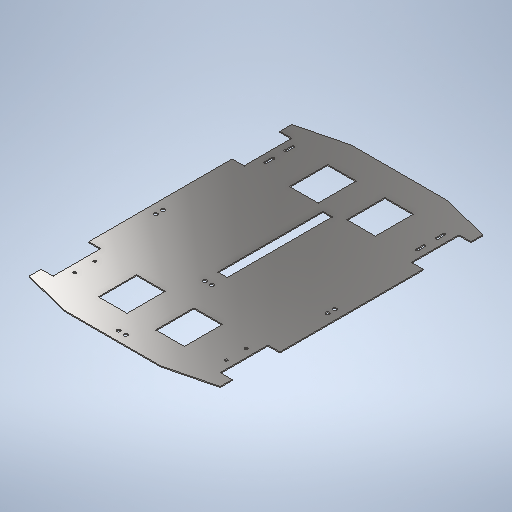
# Autodesk Inventor part: chassis
Saved by Autodesk Inventor 2026.1 (Build 301233020, 233B)
## iProperties
Created: 2026-01-22
Part Number: chassis
Material: Steel, Mild
Document SubType Name: Modeling
Designer: user
Density: 7.85 g/cm^3
Appearance: Semi-Polished
Mass: 3211.32 g
Surface Area: 4154.01 cm^2
Volume: 409.085 cm^3
Author: user
Autodesk Inventor part; units mm, degrees
ref_plane "YZ Plane" through (0, 0, 0) normal (1, 0, 0) x (0, 1, 0)
ref_plane "XZ Plane" through (0, 0, 0) normal (0, 1, 0) x (-1, 0, 0)
sketch "Sketch1" plane through (0, 0, 0) normal (0, 1, 0) x (-1, 0, 0)
  line L0 (-200, 300) -> (200, 300)
  line L1 (200, 300) -> (200, -300)
  line L2 (200, -300) -> (-200, -300)
  line L3 (-200, -300) -> (-200, 300)
  line L4 (-200, 300) -> (200, -300) construction
  line L5 (200, 300) -> (-200, -300) construction
  point P0 (0, 0)
  dimension "d0" = 400
  dimension "d1" = 600
  constraints: 12 end point, 2 midpoint, 2 parallel, 1 horizontal, 1 perpendicular
  measures "d0" distance of L1.end L2.end
  measures "d1" distance of L0.end L1.end
extrude "Extrusion1" add sketch "Sketch1" along normal blind 2
sketch "Sketch2" plane through (0, 2, 0) normal (0, 1, 0) x (1, 0, 0)
  line L0 (200, 300) -> (-200, 300) projected
  line L1 (-200, 300) -> (-200, 275)
  line L2 (-200, 300) -> (-200, -300) projected
  line L3 (-200, 300) -> (-100, 300)
  line L4 (-100, 300) -> (-200, 275)
  line L5 (-200, 275) -> (-200, 250)
  line L6 (-200, 250) -> (-175, 250)
  line L7 (-175, 250) -> (-175, 150)
  line L8 (-175, 150) -> (-200, 150)
  line L9 (-200, 250) -> (-200, 150)
  line L10 (0, 250) -> (0, 74.4907)
  line L11 (-155.9773, 0) -> (157.8952, 0)
  line L12 (-200, 300) -> (200, 300)
  line L13 (200, 300) -> (200, -300)
  line L14 (100, 300) -> (200, 275)
  line L15 (200, 250) -> (175, 250)
  line L16 (175, 250) -> (175, 150)
  line L17 (175, 150) -> (200, 150)
  line L18 (200, -300) -> (-200, -300)
  line L19 (-200, -300) -> (-200, -275)
  line L20 (-200, -300) -> (-100, -300)
  line L21 (-100, -300) -> (-200, -275)
  line L22 (-200, -275) -> (-200, -250)
  line L23 (-200, -250) -> (-175, -250)
  line L24 (-175, -250) -> (-175, -150)
  line L25 (-175, -150) -> (-200, -150)
  line L26 (-200, -250) -> (-200, -150)
  line L27 (175, -250) -> (175, -150)
  line L28 (175, -150) -> (200, -150)
  line L29 (200, -300) -> (200, 300)
  line L30 (200, -250) -> (175, -250)
  line L31 (100, -300) -> (200, -275)
  line L32 (-200, -300) -> (200, -300)
  point P0 (0, 0)
  dimension "d4" = 25
  dimension "d5" = 100
  dimension "d6" = 25
  dimension "d7" = 25
  dimension "d8" = 100
  constraints: 62 end point, 26 symmetric about line, 13 point on line, 3 perpendicular, 1 collinear, 1 horizontal, 1 vertical
  measures "d4" distance of L0.end L1.end
  measures "d5" distance of L0.end L3.end
  measures "d6" distance of L1.end L5.end
  measures "d7" distance of L5.end L6.end
  measures "d8" distance of L6.end L7.end
extrude "Extrusion2" cut sketch "Sketch2" against normal blind 2 contours L13 L14 L0 | L4 L1 L0 | L13 L17 L16 L15 | L6 L7 L8 L2 | L13 L30 L27 L28 | L25 L24 L23 L2 | L13 L18 L31 | L21 L18 L2
sketch "Sketch3" plane through (0, 2, 0) normal (0, 1, 0) x (1, 0, 0)
  line L0 (-175, 250) -> (-200, 250) projected
  line L1 (-175, 250) -> (-175, 200)
  line L2 (-175, 150) -> (-175, 250) projected
  line L3 (175, 250) -> (200, 250) projected
  line L4 (175, 250) -> (175, 200)
  line L5 (175, 250) -> (175, 150) projected
  line L6 (175, 200) -> (-175, 200)
  line L7 (-175, -150) -> (-175, -251.235)
  line L8 (-175, -251.235) -> (-175, -201.235)
  line L9 (-175, -150) -> (-175, -250) projected
  line L10 (-175, -201.235) -> (175, -201.235)
  line L11 (-175, 200) -> (-165, 200)
  line L12 (-165, 200) -> (-165, 227.5)
  line L13 (-165, 227.5) -> (-152, 227.5)
  line L14 (-152, 227.5) -> (-152, 172.5)
  line L15 (-152, 172.5) -> (-165, 172.5)
  line L16 (-165, 172.5) -> (-165, 200)
  line L17 (0, 46.6917) -> (0, -57.1112)
  line L18 (0, 0) -> (63.947, 0)
  line L19 (63.947, 0) -> (-44.9417, 0)
  line L20 (165, 200) -> (165, 227.5)
  line L21 (165, 227.5) -> (152, 227.5)
  line L22 (152, 227.5) -> (152, 172.5)
  line L23 (152, 172.5) -> (165, 172.5)
  line L24 (165, 172.5) -> (165, 200)
  line L25 (-165, -200) -> (-165, -227.5)
  line L26 (-165, -227.5) -> (-152, -227.5)
  line L27 (-152, -227.5) -> (-152, -172.5)
  line L28 (-152, -172.5) -> (-165, -172.5)
  line L29 (-165, -172.5) -> (-165, -200)
  line L30 (152, -227.5) -> (152, -172.5)
  line L31 (152, -172.5) -> (165, -172.5)
  line L32 (165, -172.5) -> (165, -200)
  line L33 (165, -200) -> (165, -227.5)
  line L34 (165, -227.5) -> (152, -227.5)
  line L35 (-165, 227.5) -> (-158.5, 227.5)
  line L36 (-158.5, 227.5) -> (-158.5, 221)
  circle A0 centre (-158.5, 221) radius 2.5
  circle A1 centre (-158.5, 179) radius 2.5
  circle A2 centre (158.5, 221) radius 2.5
  circle A3 centre (158.5, 179) radius 2.5
  circle A4 centre (158.5, -179) radius 2.5
  circle A5 centre (158.5, -221) radius 2.5
  circle A6 centre (-158.5, -179) radius 3
  circle A7 centre (-158.5, -221) radius 3
  dimension "d11" = 50
  dimension "d12" = 50
  dimension "d13" = 50
  dimension "d14" = 10
  dimension "d15" = 27.5
  dimension "d16" = 13
  dimension "d17" = 55
  dimension "d18" = 6.5
  dimension "d19" = 5
  dimension "d110" = 6
  dimension "d111" = 6
  constraints: 64 end point, 20 symmetric about line, 8 centre point, 8 perpendicular, 7 point on line, 3 midpoint, 2 vertical, 1 coincident, 1 horizontal, 5 other
  measures "d11" distance of L0.start L1.end
  measures "d12" distance of L3.start L4.end
  measures "d13" distance of L7.end L8.end
  measures "d14" distance of L1.end L11.end
  measures "d15" distance of L11.end L12.end
  measures "d16" distance of L12.end L13.end
  measures "d17" distance of L13.end L14.end
  measures "d18" distance of L35.end L36.end
  measures "d19" diameter of A0
  measures "d110" diameter of A6
  measures "d111" diameter of A7
extrude "Extrusion3" cut sketch "Sketch3" against normal blind 2 contours A0 | A1 | A2 | A3 | A4 | A5
sketch "Sketch8" plane through (0, 2, 0) normal (0, 1, 0) x (1, 0, 0)
  circle A0 centre (-158.5, 179) radius 2.5 projected
  arc A1 (-161, 179) -> (-156, 179) centre (-158.5, 179) ccw
  line L0 (-161, 179) -> (-161, 194)
  arc A2 (-156, 194) -> (-161, 194) centre (-158.5, 194) ccw
  line L1 (-156, 194) -> (-156, 179)
  line L2 (-175, 150) -> (-175, 250) projected
  line L3 (-175, 250) -> (-175, 200)
  line L4 (-175, 200) -> (-70.1244, 199)
  arc A3 (-161, 221.0527) -> (-156, 221.0527) centre (-158.5, 221.0527) ccw
  line L5 (-161, 221.0527) -> (-161, 236.0527)
  arc A4 (-156, 236.0527) -> (-161, 236.0527) centre (-158.5, 236.0527) ccw
  line L6 (-156, 236.0527) -> (-156, 221.0527)
  line L7 (0, 245.5102) -> (0, 190.0088)
  arc A5 (156, 179) -> (161, 179) centre (158.5, 179) ccw
  line L8 (161, 179) -> (161, 194)
  arc A6 (161, 194) -> (156, 194) centre (158.5, 194) ccw
  line L9 (156, 194) -> (156, 179)
  line L10 (161, 221.0527) -> (161, 236.0527)
  line L11 (156, 236.0527) -> (156, 221.0527)
  arc A7 (161, 236.0527) -> (156, 236.0527) centre (158.5, 236.0527) ccw
  arc A8 (156, 221.0527) -> (161, 221.0527) centre (158.5, 221.0527) ccw
  point P0 (0, 0)
  point P1 (-156, 179)
  dimension "d47" = 15
  dimension "d48" = 50
  dimension "d49" = 15
  constraints: 22 end point, 16 point on circle, 12 symmetric about line, 8 centre point, 7 tangent, 3 vertical, 1 coincident, 1 midpoint, 4 other
  measures "d47" distance of L0.start L0.end
  measures "d48" distance of L2.end L3.end
  measures "d49" distance of L5.start L5.end
extrude "Extrusion7" cut sketch "Sketch8" against normal blind 2
mirror "Mirror2" about plane through (0, 0, 0) normal (1, 0, 0)
ref_plane "Work Plane2" through (-100, 0, 190) normal (0, 0, 1) x (1, 0, 0)
mirror "Mirror4" about plane through (-100, 0, 190) normal (0, 0, 1) of "Mirror2"
sketch "Sketch11" plane through (0, 2, 0) normal (0, 1, 0) x (1, 0, 0)
  line L0 (-200, 150) -> (-200, -150) projected
  line L1 (-200, 0) -> (-200, -30)
  line L2 (-200, -30) -> (-170, -30)
  line L3 (-170, -30) -> (-170, 0)
  line L4 (-170, 0) -> (-170, -15)
  line L5 (-170, -15) -> (-180, -15)
  line L6 (-180, -15) -> (-179, -15)
  line L7 (-180, -15) -> (-180, -14)
  line L8 (-180, -15) -> (-180, -16)
  circle A0 centre (-180, -15) radius 4
  circle A1 centre (-180, -30) radius 4
  line L9 (0, -7.5) -> (0, -36.2272)
  circle A2 centre (180, -15) radius 4
  circle A3 centre (180, -30) radius 4
  point P0 (0, 0)
  dimension "d65" = 30
  dimension "d66" = 30
  dimension "d67" = 10
  dimension "d68" = 1
  dimension "d70" = 1
  dimension "d71" = 1
  dimension "d74" = 8
  dimension "d75" = 8
  dimension "d108" = 15
  constraints: 18 end point, 4 centre point, 3 perpendicular, 3 vertical, 2 midpoint, 2 point on line, 2 symmetric about line, 2 other
  measures "d65" distance of L1.start L1.end
  measures "d66" distance of L1.end L2.end
  measures "d67" distance of L4.end L5.end
  measures "d68" distance of L5.end L6.end
  measures "d70" distance of L5.end L7.end
  measures "d71" distance of L5.end L8.end
  measures "d74" diameter of A0
  measures "d75" diameter of A1
  measures "d108" distance of A1.centre A0.centre
extrude "Extrusion9" cut sketch "Sketch11" against normal blind 2
sketch "Sketch12" plane through (0, 2, 0) normal (0, 1, 0) x (1, 0, 0)
  line L0 (-200, -150) -> (-175, -150) projected
  line L1 (-200, -150) -> (-200, -200)
  line L2 (-200, -200) -> (258.9197, -200)
  line L3 (0, -200) -> (-30, -200)
  line L4 (-30, -200) -> (-30, -150)
  line L5 (-90, -150) -> (-90, -250)
  line L6 (-30, -250) -> (-30, -200)
  line L7 (-90, -240) -> (-30, -240)
  line L8 (-30, -240) -> (-30, -160)
  line L9 (-30, -160) -> (-90, -160)
  line L10 (-90, -160) -> (-90, -240)
  line L11 (-90, -240) -> (-30, -160) construction
  line L12 (-30, -240) -> (-90, -160) construction
  point P0 (0, 0)
  point P1 (-60, -200)
  point P2 (-90, -240)
  point P3 (-30, -240)
  point P4 (-30, -160)
  point P5 (-90, -160)
  dimension "d78" = 50
  dimension "d79" = 30
  dimension "d81" = 60
  dimension "d82" = 100
  dimension "d107" = 80
  constraints: 24 end point, 4 perpendicular, 3 point on line, 2 midpoint, 2 parallel, 1 horizontal, 1 vertical
  measures "d78" distance of L0.start L1.end
  measures "d79" distance of L3.start L3.end
  measures "d81" distance of L4.end L5.start
  measures "d82" distance of L5.start L5.end
  measures "d107" distance of L8.end L7.end
extrude "Extrusion10" cut sketch "Sketch12" against normal blind 10
mirror "Mirror5" about plane through (0, 0, 0) normal (1, 0, 0) of "Extrusion10"
mirror "Mirror6" about plane through (0, 0, 0) normal (0, 0, 1) of "Extrusion10", "Mirror5"
sketch "Sketch13" plane through (0, 2, 0) normal (0, 1, 0) x (1, 0, 0)
  line L0 (-100, -300) -> (100, -300) projected
  line L1 (0, -300) -> (15, -300)
  line L2 (15, -300) -> (15, -270)
  line L3 (15, -270) -> (-15, -270)
  line L4 (-15, -270) -> (-15, -300)
  line L5 (0, -300) -> (-15, -300)
  line L6 (-15, -270) -> (-15, -280)
  line L7 (-15, -280) -> (-7.5, -280)
  line L8 (-7.5, -280) -> (7.5, -280)
  circle A0 centre (-7.5, -280) radius 4
  circle A1 centre (7.5, -280) radius 4
  point P0 (0, 0)
  dimension "d85" = 15
  dimension "d86" = 30
  dimension "d87" = 30
  dimension "d88" = 10
  dimension "d90" = 15
  dimension "d91" = 8
  dimension "d92" = 8
  dimension "d114" = 7.5
  constraints: 16 end point, 4 perpendicular, 4 point on line, 2 centre point, 2 coincident, 1 collinear, 1 midpoint
  measures "d85" distance of L1.start L1.end
  measures "d86" distance of L1.end L2.end
  measures "d87" distance of L2.end L3.end
  measures "d88" distance of L3.end L6.end
  measures "d90" distance of L7.end L8.end
  measures "d91" diameter of A0
  measures "d92" diameter of A1
  measures "d114" distance of L6.end A0.centre
extrude "Extrusion11" cut sketch "Sketch13" against normal blind 10 contours A0 L8 L7 | L7 L8 A0 | A1
sketch "Sketch14" plane through (0, 2, 0) normal (0, 1, 0) x (1, 0, 0)
  circle A0 centre (7.5, -280) radius 4 projected
  line L0 (7.5, -280) -> (7.5, -100)
  circle A1 centre (7.5, -100) radius 4
  line L1 (7.5, -100) -> (-7.5, -100)
  circle A2 centre (-7.5, -100) radius 4
  point P0 (0, 0)
  dimension "d95" = 180
  dimension "d96" = 8
  dimension "d97" = 15
  dimension "d98" = 8
  constraints: 4 end point, 2 centre point, 2 coincident, 1 horizontal, 1 vertical
  measures "d95" distance of L0.start L0.end
  measures "d96" diameter of A1
  measures "d97" distance of L1.start L1.end
  measures "d98" diameter of A2
extrude "Extrusion12" cut sketch "Sketch14" against normal blind 10 contours A1 L1 L0 | L0 L1 A1 | A2
sketch "Sketch15" plane through (0, 2, 0) normal (0, 1, 0) x (1, 0, 0)
  line L0 (-10, -70) -> (10, -70)
  line L1 (10, -70) -> (10, 70)
  line L2 (10, 70) -> (-10, 70)
  line L3 (-10, 70) -> (-10, -70)
  line L4 (-10, -70) -> (10, 70) construction
  line L5 (10, -70) -> (-10, 70) construction
  line L6 (-10, 70) -> (-10, 150)
  line L7 (-10, 150) -> (10, 150)
  line L8 (10, 150) -> (10, 70)
  point P0 (0, 0)
  dimension "d101" = 20
  dimension "d102" = 140
  dimension "d103" = 80
  constraints: 18 end point, 3 perpendicular, 2 midpoint, 2 parallel, 1 horizontal, 1 vertical
  measures "d101" distance of L2.end L1.end
  measures "d102" distance of L1.end L0.end
  measures "d103" distance of L2.end L6.end
extrude "Extrusion13" cut sketch "Sketch15" against normal blind 10
extrude "Extrusion14" cut sketch "Sketch3" against normal blind 10 contours A6 | A7
mirror "Mirror7" about plane through (0, 0, 0) normal (1, 0, 0) of "Extrusion14"
mirror "Mirror8" about plane through (0, 0, 0) normal (0, 0, 1) of "Extrusion14", "Mirror7"
ref_plane "Work Plane1" through (0, 0, 0) normal (1, 0, 0) x (0, 1, 0)
ref_plane "Work Plane3" through (0, 0, 380) normal (-1, 0, 0) x (0, 1, 0)
ref_plane "Work Plane4" through (0, 0, 380) normal (-1, 0, 0) x (0, 1, 0)
body "Solid1"
